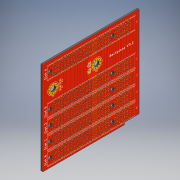
# Autodesk Inventor part: Backplane_PCB
Saved by Autodesk Inventor 2018 (Build 220112000, 112)
## iProperties
Created: 2018-10-18
Part Number: Backplane_PCB
Material: Epoxy Resin
Document SubType Name: Modeling
Designer: Bradley
Density: 1.14 g/cm^3
Appearance: Smooth - Dark Gray
Author: Bradley
Autodesk Inventor part; units mm, degrees
ref_plane "YZ Plane" through (0, 0, 0) normal (1, 0, 0) x (0, 1, 0)
ref_plane "XZ Plane" through (0, 0, 0) normal (0, 1, 0) x (-1, 0, 0)
ref_plane "XY Plane" through (0, 0, 0) normal (0, 0, 1) x (1, 0, 0)
sketch "Sketch11" plane through (0, 0, 0) normal (1, 0, 0) x (0, 1, 0)
  line L0 (-41.4, 41.6) -> (-32, 41.6)
  line L1 (-32, 41.6) -> (-32, 43)
  line L2 (-32, 43) -> (32, 43)
  line L3 (32, 43) -> (32, 41.6)
  line L4 (32, 41.6) -> (41.4, 41.6)
  line L5 (41.4, 41.6) -> (41.4, -41.6)
  line L6 (41.4, -41.6) -> (32, -41.6)
  line L7 (32, -41.6) -> (32, -43)
  line L8 (32, -43) -> (-32, -43)
  line L9 (-32, -43) -> (-32, -41.6)
  line L10 (-32, -41.6) -> (-41.4, -41.6)
  line L11 (-41.4, -41.6) -> (-41.4, 41.6)
  line L12 (41.4, 17) -> (-21, 17)
  line L13 (-21, 17) -> (-21, -43)
  point P0 (0, 0)
  point P1 (0, 43)
  point P2 (-41.4, 0)
  dimension "d86" = 83.2
  dimension "d87" = 9.4
  dimension "d88" = 82.8
  dimension "d89" = 86
  dimension "d149" = 21
  dimension "d150" = 17
  constraints: 28 end point, 9 perpendicular, 7 point on line, 3 collinear, 2 horizontal, 2 midpoint, 1 horizontal alignment, 1 vertical, 1 vertical alignment
  measures "d86" distance of L4.end L5.end
  measures "d87" distance of L3.end L4.end
  measures "d88" distance between parallel lines of L11 L5
  measures "d89" distance between parallel lines of L8 L2
  measures "d149" distance from line of point (0, 0) L13
  measures "d150" distance from line of point (0, 0) L12
extrude "Extrusion3" add sketch "Sketch11" along normal mid plane 1 contours L13 L12 L5 L6 L7 L8
fillet "Fillet2" radius 0.5 6 edges at (0, 32, -43) (0, 32, -41.6) (0, 41.4, -41.6) (0, -21, 17) (0, -21, -43) (0, 41.4, 17)
sketch "Sketch19" plane through (0.5, 0, 0) normal (1, 0, 0) x (0, 0, -1)
  line L0 (-17, -21.0036) -> (-17, 41.4036) construction
  line L1 (-17, 41.4036) -> (43, 41.4036) construction
  line L2 (43, 41.4036) -> (43, -21.0036) construction
  line L3 (43, -21.0036) -> (-17, -21.0036) construction
  line L4 (-17, 40.9) -> (-17, -20.5) projected
  line L5 (43, -20.5) -> (43, 31.5) projected
  point P0 (0, 0)
  point P1 (-17, 10.2)
  constraints: 2 collinear, 2 midpoint, 2 other
decal "Decal5"
sketch "Sketch20" plane through (-0.5, 0, 0) normal (-1, 0, 0) x (0, 0, 1)
  line L0 (17, 41.4036) -> (17, -21.0036) construction
  line L1 (17, -21.0036) -> (-43, -21.0036) construction
  line L2 (-43, -21.0036) -> (-43, 41.4036) construction
  line L3 (-43, 41.4036) -> (17, 41.4036) construction
  line L4 (17, -20.5) -> (17, 40.9) projected
  line L5 (-43, 31.5) -> (-43, -20.5) projected
  point P0 (0, 0)
  point P1 (17, 10.2)
  constraints: 2 collinear, 2 midpoint, 2 other
decal "Decal6"
sketch "Sketch14" plane through (0.5, 0, 0) normal (1, 0, 0) x (0, 0, -1)
  point P0 (0, 0)
  point P1 (0, -14)
  point P2 (0, 14)
  constraints: 2 other
hole "Hole7" at (0.5, -14, 0) at (0.5, 14, 0) direction (-1, 0, 0) diameter 3.3 end through all
sketch "Sketch15" plane through (0.5, 0, 0) normal (1, 0, 0) x (0, 0, -1)
  point P0 (0, 0)
  point P1 (37.5, 24)
  point P2 (37.5, -16.15)
  point P3 (28.5, 24)
  point P4 (28.5, -16.15)
  point P5 (19.5, 24)
  point P6 (19.5, -16.15)
  point P7 (10.5, 24)
  point P8 (10.5, -16.15)
  point P9 (-10.5, 24)
  point P10 (-10.5, -16.15)
  constraints: 10 other
hole "Hole8" at (0.5, 24, -37.5) at (0.5, -16.15, -37.5) at (0.5, 24, -28.5) at (0.5, -16.15, -28.5) at (0.5, 24, -19.5) at (0.5, -16.15, -19.5) at (0.5, 24, -10.5) at (0.5, -16.15, -10.5) at (0.5, 24, 10.5) at (0.5, -16.15, 10.5) direction (-1, 0, 0) diameter 2.35 end through all
sketch "Sketch16" plane through (0.5, 0, 0) normal (1, 0, 0) x (0, 0, -1)
  point P0 (0, 0)
  point P1 (40.75, 0.65)
  point P2 (36.25, 25.65)
  point P3 (34.25, 26.65)
  point P4 (40.75, 26.65)
  point P5 (38.75, 25.65)
  point P6 (36.25, 27.65)
  point P7 (34.25, 28.65)
  point P8 (40.75, 28.65)
  point P9 (38.75, 27.65)
  point P10 (36.25, 29.65)
  point P11 (34.25, 30.65)
  point P12 (40.75, 30.65)
  point P13 (38.75, 29.65)
  point P14 (36.25, 31.65)
  point P15 (34.25, 32.65)
  point P16 (40.75, 32.65)
  point P17 (38.75, 31.65)
  point P18 (36.25, 33.65)
  point P19 (34.25, 34.65)
  point P20 (40.75, 34.65)
  point P21 (38.75, 33.65)
  point P22 (36.25, 35.65)
  point P23 (38.75, 35.65)
  point P24 (34.25, 22.65)
  point P25 (40.75, 22.65)
  point P26 (38.75, 21.65)
  point P27 (36.25, 21.65)
  point P28 (34.25, 20.65)
  point P29 (40.75, 20.65)
  point P30 (38.75, 19.65)
  point P31 (36.25, 19.65)
  point P32 (34.25, 18.65)
  point P33 (40.75, 18.65)
  point P34 (38.75, 17.65)
  point P35 (36.25, 17.65)
  point P36 (34.25, 16.65)
  point P37 (40.75, 16.65)
  point P38 (38.75, 15.65)
  point P39 (36.25, 15.65)
  point P40 (34.25, 14.65)
  point P41 (40.75, 14.65)
  point P42 (38.75, 13.65)
  point P43 (36.25, 13.65)
  point P44 (34.25, 12.65)
  point P45 (40.75, 12.65)
  point P46 (38.75, 11.65)
  point P47 (36.25, 11.65)
  point P48 (34.25, 10.65)
  point P49 (40.75, 10.65)
  point P50 (38.75, 9.65)
  point P51 (36.25, 9.65)
  point P52 (34.25, 8.65)
  point P53 (40.75, 8.65)
  point P54 (38.75, 7.65)
  point P55 (36.25, 7.65)
  point P56 (34.25, 6.65)
  point P57 (40.75, 6.65)
  point P58 (38.75, 5.65)
  point P59 (36.25, 5.65)
  point P60 (34.25, 4.65)
  point P61 (40.75, 4.65)
  point P62 (38.75, 3.65)
  point P63 (36.25, 3.65)
  point P64 (34.25, 2.65)
  point P65 (40.75, 2.65)
  point P66 (38.75, 1.65)
  point P67 (36.25, 1.65)
  point P68 (34.25, 0.65)
  point P69 (38.75, -0.35)
  point P70 (36.25, -0.35)
  point P71 (34.25, -1.35)
  point P72 (40.75, -1.35)
  point P73 (38.75, -2.35)
  point P74 (36.25, -2.35)
  point P75 (34.25, -3.35)
  point P76 (40.75, -3.35)
  point P77 (38.75, -4.35)
  point P78 (36.25, -4.35)
  point P79 (34.25, -5.35)
  point P80 (40.75, -5.35)
  point P81 (38.75, -6.35)
  point P82 (36.25, -6.35)
  point P83 (34.25, -7.35)
  point P84 (40.75, -7.35)
  point P85 (38.75, -8.35)
  point P86 (36.25, -8.35)
  point P87 (34.25, -9.35)
  point P88 (40.75, -9.35)
  point P89 (38.75, -10.35)
  point P90 (36.25, -10.35)
  point P91 (34.25, -11.35)
  point P92 (40.75, -11.35)
  point P93 (38.75, -12.35)
  point P94 (36.25, -12.35)
  point P95 (34.25, -13.35)
  point P96 (40.75, -13.35)
  point P97 (38.75, -14.35)
  point P98 (36.25, -14.35)
  point P99 (27.25, 25.65)
  point P100 (25.25, 26.65)
  point P101 (31.75, 26.65)
  point P102 (29.75, 25.65)
  point P103 (27.25, 27.65)
  point P104 (25.25, 28.65)
  point P105 (31.75, 28.65)
  point P106 (29.75, 27.65)
  point P107 (27.25, 29.65)
  point P108 (25.25, 30.65)
  point P109 (31.75, 30.65)
  point P110 (29.75, 29.65)
  point P111 (27.25, 31.65)
  point P112 (25.25, 32.65)
  point P113 (31.75, 32.65)
  point P114 (29.75, 31.65)
  point P115 (27.25, 33.65)
  point P116 (25.25, 34.65)
  point P117 (31.75, 34.65)
  point P118 (29.75, 33.65)
  point P119 (27.25, 35.65)
  point P120 (29.75, 35.65)
  point P121 (25.25, 22.65)
  point P122 (31.75, 22.65)
  point P123 (29.75, 21.65)
  point P124 (27.25, 21.65)
  point P125 (25.25, 20.65)
  point P126 (31.75, 20.65)
  point P127 (29.75, 19.65)
  point P128 (27.25, 19.65)
  point P129 (25.25, 18.65)
  point P130 (31.75, 18.65)
  point P131 (29.75, 17.65)
  point P132 (27.25, 17.65)
  point P133 (25.25, 16.65)
  point P134 (31.75, 16.65)
  point P135 (29.75, 15.65)
  point P136 (27.25, 15.65)
  point P137 (25.25, 14.65)
  point P138 (31.75, 14.65)
  point P139 (29.75, 13.65)
  point P140 (27.25, 13.65)
  point P141 (25.25, 12.65)
  point P142 (31.75, 12.65)
  point P143 (29.75, 11.65)
  point P144 (27.25, 11.65)
  point P145 (25.25, 10.65)
  point P146 (31.75, 10.65)
  point P147 (29.75, 9.65)
  point P148 (27.25, 9.65)
  point P149 (25.25, 8.65)
  point P150 (31.75, 8.65)
  point P151 (29.75, 7.65)
  point P152 (27.25, 7.65)
  point P153 (25.25, 6.65)
  point P154 (31.75, 6.65)
  point P155 (29.75, 5.65)
  point P156 (27.25, 5.65)
  point P157 (25.25, 4.65)
  point P158 (31.75, 4.65)
  point P159 (29.75, 3.65)
  point P160 (27.25, 3.65)
  point P161 (25.25, 2.65)
  point P162 (31.75, 2.65)
  point P163 (29.75, 1.65)
  point P164 (27.25, 1.65)
  point P165 (25.25, 0.65)
  point P166 (31.75, 0.65)
  point P167 (29.75, -0.35)
  point P168 (27.25, -0.35)
  point P169 (25.25, -1.35)
  point P170 (31.75, -1.35)
  point P171 (29.75, -2.35)
  point P172 (27.25, -2.35)
  point P173 (25.25, -3.35)
  point P174 (31.75, -3.35)
  point P175 (29.75, -4.35)
  point P176 (27.25, -4.35)
  point P177 (25.25, -5.35)
  point P178 (31.75, -5.35)
  point P179 (29.75, -6.35)
  point P180 (27.25, -6.35)
  point P181 (25.25, -7.35)
  point P182 (31.75, -7.35)
  point P183 (29.75, -8.35)
  point P184 (27.25, -8.35)
  point P185 (25.25, -9.35)
  point P186 (31.75, -9.35)
  point P187 (29.75, -10.35)
  point P188 (27.25, -10.35)
  point P189 (25.25, -11.35)
  point P190 (31.75, -11.35)
  point P191 (29.75, -12.35)
  point P192 (27.25, -12.35)
  point P193 (25.25, -13.35)
  point P194 (31.75, -13.35)
  point P195 (29.75, -14.35)
  point P196 (27.25, -14.35)
  point P197 (18.25, 25.65)
  point P198 (16.25, 26.65)
  point P199 (22.75, 26.65)
  constraints: 490 other
hole "Hole9" at (0.5, 0.65, -40.75) at (0.5, 25.65, -36.25) at (0.5, 26.65, -34.25) at (0.5, 26.65, -40.75) at (0.5, 25.65, -38.75) at (0.5, 27.65, -36.25) at (0.5, 28.65, -34.25) at (0.5, 28.65, -40.75) at (0.5, 27.65, -38.75) at (0.5, 29.65, -36.25) at (0.5, 30.65, -34.25) at (0.5, 30.65, -40.75) at (0.5, 29.65, -38.75) at (0.5, 31.65, -36.25) at (0.5, 32.65, -34.25) at (0.5, 32.65, -40.75) at (0.5, 31.65, -38.75) at (0.5, 33.65, -36.25) at (0.5, 34.65, -34.25) at (0.5, 34.65, -40.75) at (0.5, 33.65, -38.75) at (0.5, 35.65, -36.25) at (0.5, 35.65, -38.75) at (0.5, 22.65, -34.25) at (0.5, 22.65, -40.75) at (0.5, 21.65, -38.75) at (0.5, 21.65, -36.25) at (0.5, 20.65, -34.25) at (0.5, 20.65, -40.75) at (0.5, 19.65, -38.75) at (0.5, 19.65, -36.25) at (0.5, 18.65, -34.25) at (0.5, 18.65, -40.75) at (0.5, 17.65, -38.75) at (0.5, 17.65, -36.25) at (0.5, 16.65, -34.25) at (0.5, 16.65, -40.75) at (0.5, 15.65, -38.75) at (0.5, 15.65, -36.25) at (0.5, 14.65, -34.25) at (0.5, 14.65, -40.75) at (0.5, 13.65, -38.75) at (0.5, 13.65, -36.25) at (0.5, 12.65, -34.25) at (0.5, 12.65, -40.75) at (0.5, 11.65, -38.75) at (0.5, 11.65, -36.25) at (0.5, 10.65, -34.25) at (0.5, 10.65, -40.75) at (0.5, 9.65, -38.75) direction (-1, 0, 0) diameter 0.7 end through all and at (0.5, 9.65, -36.25) (0.5, 8.65, -34.25) (0.5, 8.65, -40.75) (0.5, 7.65, -38.75) (0.5, 7.65, -36.25) (0.5, 6.65, -34.25) (0.5, 6.65, -40.75) (0.5, 5.65, -38.75) (0.5, 5.65, -36.25) (0.5, 4.65, -34.25) (0.5, 4.65, -40.75) (0.5, 3.65, -38.75) (0.5, 3.65, -36.25) (0.5, 2.65, -34.25) (0.5, 2.65, -40.75) (0.5, 1.65, -38.75) (0.5, 1.65, -36.25) (0.5, 0.65, -34.25) (0.5, -0.35, -38.75) (0.5, -0.35, -36.25) (0.5, -1.35, -34.25) (0.5, -1.35, -40.75) (0.5, -2.35, -38.75) (0.5, -2.35, -36.25) (0.5, -3.35, -34.25) (0.5, -3.35, -40.75) (0.5, -4.35, -38.75) (0.5, -4.35, -36.25) (0.5, -5.35, -34.25) (0.5, -5.35, -40.75) (0.5, -6.35, -38.75) (0.5, -6.35, -36.25) (0.5, -7.35, -34.25) (0.5, -7.35, -40.75) (0.5, -8.35, -38.75) (0.5, -8.35, -36.25) (0.5, -9.35, -34.25) (0.5, -9.35, -40.75) (0.5, -10.35, -38.75) (0.5, -10.35, -36.25) (0.5, -11.35, -34.25) (0.5, -11.35, -40.75) (0.5, -12.35, -38.75) (0.5, -12.35, -36.25) (0.5, -13.35, -34.25) (0.5, -13.35, -40.75) (0.5, -14.35, -38.75) (0.5, -14.35, -36.25) (0.5, 25.65, -27.25) (0.5, 26.65, -25.25) (0.5, 26.65, -31.75) (0.5, 25.65, -29.75) (0.5, 27.65, -27.25) (0.5, 28.65, -25.25) (0.5, 28.65, -31.75) (0.5, 27.65, -29.75) (0.5, 29.65, -27.25) (0.5, 30.65, -25.25) (0.5, 30.65, -31.75) (0.5, 29.65, -29.75) (0.5, 31.65, -27.25) (0.5, 32.65, -25.25) (0.5, 32.65, -31.75) (0.5, 31.65, -29.75) (0.5, 33.65, -27.25) (0.5, 34.65, -25.25) (0.5, 34.65, -31.75) (0.5, 33.65, -29.75) (0.5, 35.65, -27.25) (0.5, 35.65, -29.75) (0.5, 22.65, -25.25) (0.5, 22.65, -31.75) (0.5, 21.65, -29.75) (0.5, 21.65, -27.25) (0.5, 20.65, -25.25) (0.5, 20.65, -31.75) (0.5, 19.65, -29.75) (0.5, 19.65, -27.25) (0.5, 18.65, -25.25) (0.5, 18.65, -31.75) (0.5, 17.65, -29.75) (0.5, 17.65, -27.25) (0.5, 16.65, -25.25) (0.5, 16.65, -31.75) (0.5, 15.65, -29.75) (0.5, 15.65, -27.25) (0.5, 14.65, -25.25) (0.5, 14.65, -31.75) (0.5, 13.65, -29.75) (0.5, 13.65, -27.25) (0.5, 12.65, -25.25) (0.5, 12.65, -31.75) (0.5, 11.65, -29.75) (0.5, 11.65, -27.25) (0.5, 10.65, -25.25) (0.5, 10.65, -31.75) (0.5, 9.65, -29.75) (0.5, 9.65, -27.25) (0.5, 8.65, -25.25) (0.5, 8.65, -31.75) (0.5, 7.65, -29.75) (0.5, 7.65, -27.25) (0.5, 6.65, -25.25) (0.5, 6.65, -31.75) (0.5, 5.65, -29.75) (0.5, 5.65, -27.25) (0.5, 4.65, -25.25) (0.5, 4.65, -31.75) (0.5, 3.65, -29.75) (0.5, 3.65, -27.25) (0.5, 2.65, -25.25) (0.5, 2.65, -31.75) (0.5, 1.65, -29.75) (0.5, 1.65, -27.25) (0.5, 0.65, -25.25) (0.5, 0.65, -31.75) (0.5, -0.35, -29.75) (0.5, -0.35, -27.25) (0.5, -1.35, -25.25) (0.5, -1.35, -31.75) (0.5, -2.35, -29.75) (0.5, -2.35, -27.25) (0.5, -3.35, -25.25) (0.5, -3.35, -31.75) (0.5, -4.35, -29.75) (0.5, -4.35, -27.25) (0.5, -5.35, -25.25) (0.5, -5.35, -31.75) (0.5, -6.35, -29.75) (0.5, -6.35, -27.25) (0.5, -7.35, -25.25) (0.5, -7.35, -31.75) (0.5, -8.35, -29.75) (0.5, -8.35, -27.25) (0.5, -9.35, -25.25) (0.5, -9.35, -31.75) (0.5, -10.35, -29.75) (0.5, -10.35, -27.25) (0.5, -11.35, -25.25) (0.5, -11.35, -31.75) (0.5, -12.35, -29.75) (0.5, -12.35, -27.25) (0.5, -13.35, -25.25) (0.5, -13.35, -31.75) (0.5, -14.35, -29.75) (0.5, -14.35, -27.25) (0.5, 25.65, -18.25) (0.5, 26.65, -16.25) (0.5, 26.65, -22.75) (0.5, 25.65, -20.75) (0.5, 27.65, -18.25) (0.5, 28.65, -16.25) (0.5, 28.65, -22.75) (0.5, 27.65, -20.75) (0.5, 29.65, -18.25) (0.5, 30.65, -16.25) (0.5, 30.65, -22.75) (0.5, 29.65, -20.75) (0.5, 31.65, -18.25) (0.5, 32.65, -16.25) (0.5, 32.65, -22.75) (0.5, 31.65, -20.75) (0.5, 33.65, -18.25) (0.5, 34.65, -16.25) (0.5, 34.65, -22.75) (0.5, 33.65, -20.75) (0.5, 35.65, -18.25) (0.5, 35.65, -20.75) (0.5, 22.65, -16.25) (0.5, 22.65, -22.75) (0.5, 21.65, -20.75) (0.5, 21.65, -18.25) (0.5, 20.65, -16.25) (0.5, 20.65, -22.75) (0.5, 19.65, -20.75) (0.5, 19.65, -18.25) (0.5, 18.65, -16.25) (0.5, 18.65, -22.75) (0.5, 17.65, -20.75) (0.5, 17.65, -18.25) (0.5, 16.65, -16.25) (0.5, 16.65, -22.75) (0.5, 15.65, -20.75) (0.5, 15.65, -18.25) (0.5, 14.65, -16.25) (0.5, 14.65, -22.75) (0.5, 13.65, -20.75) (0.5, 13.65, -18.25) (0.5, 12.65, -16.25) (0.5, 12.65, -22.75) (0.5, 11.65, -20.75) (0.5, 11.65, -18.25) (0.5, 10.65, -16.25) (0.5, 10.65, -22.75) (0.5, 9.65, -20.75) (0.5, 9.65, -18.25) (0.5, 8.65, -16.25) (0.5, 8.65, -22.75) (0.5, 7.65, -20.75) (0.5, 7.65, -18.25) (0.5, 6.65, -16.25) (0.5, 6.65, -22.75) (0.5, 5.65, -20.75) (0.5, 5.65, -18.25) (0.5, 4.65, -16.25) (0.5, 4.65, -22.75) (0.5, 3.65, -20.75) (0.5, 3.65, -18.25) (0.5, 2.65, -16.25) (0.5, 2.65, -22.75) (0.5, 1.65, -20.75) (0.5, 1.65, -18.25) (0.5, 0.65, -16.25) (0.5, 0.65, -22.75) (0.5, -0.35, -20.75) (0.5, -0.35, -18.25) (0.5, -1.35, -16.25) (0.5, -1.35, -22.75) (0.5, -2.35, -20.75) (0.5, -2.35, -18.25) (0.5, -3.35, -16.25) (0.5, -3.35, -22.75) (0.5, -4.35, -20.75) (0.5, -4.35, -18.25) (0.5, -5.35, -16.25) (0.5, -5.35, -22.75) (0.5, -6.35, -20.75) (0.5, -6.35, -18.25) (0.5, -7.35, -16.25) (0.5, -7.35, -22.75) (0.5, -8.35, -20.75) (0.5, -8.35, -18.25) (0.5, -9.35, -16.25) (0.5, -9.35, -22.75) (0.5, -10.35, -20.75) (0.5, -10.35, -18.25) (0.5, -11.35, -16.25) (0.5, -11.35, -22.75) (0.5, -12.35, -20.75) (0.5, -12.35, -18.25) (0.5, -13.35, -16.25) (0.5, -13.35, -22.75) (0.5, -14.35, -20.75) (0.5, -14.35, -18.25) (0.5, 25.65, -9.25) (0.5, 26.65, -7.25) (0.5, 26.65, -13.75) (0.5, 25.65, -11.75) (0.5, 27.65, -9.25) (0.5, 28.65, -7.25) (0.5, 28.65, -13.75) (0.5, 27.65, -11.75) (0.5, 29.65, -9.25) (0.5, 30.65, -7.25) (0.5, 30.65, -13.75) (0.5, 29.65, -11.75) (0.5, 31.65, -9.25) (0.5, 32.65, -7.25) (0.5, 32.65, -13.75) (0.5, 31.65, -11.75) (0.5, 33.65, -9.25) (0.5, 34.65, -7.25) (0.5, 34.65, -13.75) (0.5, 33.65, -11.75) (0.5, 35.65, -9.25) (0.5, 35.65, -11.75) (0.5, 22.65, -7.25) (0.5, 22.65, -13.75) (0.5, 21.65, -11.75) (0.5, 21.65, -9.25) (0.5, 20.65, -7.25) (0.5, 20.65, -13.75) (0.5, 19.65, -11.75) (0.5, 19.65, -9.25) (0.5, 18.65, -7.25) (0.5, 18.65, -13.75) (0.5, 17.65, -11.75) (0.5, 17.65, -9.25) (0.5, 16.65, -7.25) (0.5, 16.65, -13.75) (0.5, 15.65, -11.75) (0.5, 15.65, -9.25) (0.5, 14.65, -7.25) (0.5, 14.65, -13.75) (0.5, 13.65, -11.75) (0.5, 13.65, -9.25) (0.5, 12.65, -7.25) (0.5, 12.65, -13.75) (0.5, 11.65, -11.75) (0.5, 11.65, -9.25) (0.5, 10.65, -7.25) (0.5, 10.65, -13.75) (0.5, 9.65, -11.75) (0.5, 9.65, -9.25) (0.5, 8.65, -7.25) (0.5, 8.65, -13.75) (0.5, 7.65, -11.75) (0.5, 7.65, -9.25) (0.5, 6.65, -7.25) (0.5, 6.65, -13.75) (0.5, 5.65, -11.75) (0.5, 5.65, -9.25) (0.5, 4.65, -7.25) (0.5, 4.65, -13.75) (0.5, 3.65, -11.75) (0.5, 3.65, -9.25) (0.5, 2.65, -7.25) (0.5, 2.65, -13.75) (0.5, 1.65, -11.75) (0.5, 1.65, -9.25) (0.5, 0.65, -7.25) (0.5, 0.65, -13.75) (0.5, -0.35, -11.75) (0.5, -0.35, -9.25) (0.5, -1.35, -7.25) (0.5, -1.35, -13.75) (0.5, -2.35, -11.75) (0.5, -2.35, -9.25) (0.5, -3.35, -7.25) (0.5, -3.35, -13.75) (0.5, -4.35, -11.75) (0.5, -4.35, -9.25) (0.5, -5.35, -7.25) (0.5, -5.35, -13.75) (0.5, -6.35, -11.75) (0.5, -6.35, -9.25) (0.5, -7.35, -7.25) (0.5, -7.35, -13.75) (0.5, -8.35, -11.75) (0.5, -8.35, -9.25) (0.5, -9.35, -7.25) (0.5, -9.35, -13.75) (0.5, -10.35, -11.75) (0.5, -10.35, -9.25) (0.5, -11.35, -7.25) (0.5, -11.35, -13.75) (0.5, -12.35, -11.75) (0.5, -12.35, -9.25) (0.5, -13.35, -7.25) (0.5, -13.35, -13.75) (0.5, -14.35, -11.75) (0.5, -14.35, -9.25) (0.5, 25.65, 11.75) (0.5, 26.65, 13.75) (0.5, 26.65, 7.25) (0.5, 25.65, 9.25) (0.5, 27.65, 11.75) (0.5, 28.65, 13.75) (0.5, 28.65, 7.25) (0.5, 27.65, 9.25) (0.5, 29.65, 11.75) (0.5, 30.65, 13.75) (0.5, 30.65, 7.25) (0.5, 29.65, 9.25) (0.5, 31.65, 11.75) (0.5, 32.65, 13.75) (0.5, 32.65, 7.25) (0.5, 31.65, 9.25) (0.5, 33.65, 11.75) (0.5, 34.65, 13.75) (0.5, 34.65, 7.25) (0.5, 33.65, 9.25) (0.5, 35.65, 11.75) (0.5, 35.65, 9.25) (0.5, 22.65, 13.75) (0.5, 22.65, 7.25) (0.5, 21.65, 9.25) (0.5, 21.65, 11.75) (0.5, 20.65, 13.75) (0.5, 20.65, 7.25) (0.5, 19.65, 9.25) (0.5, 19.65, 11.75) (0.5, 18.65, 13.75) (0.5, 18.65, 7.25) (0.5, 17.65, 9.25) (0.5, 17.65, 11.75) (0.5, 16.65, 13.75) (0.5, 16.65, 7.25) (0.5, 15.65, 9.25) (0.5, 15.65, 11.75) (0.5, 14.65, 13.75) (0.5, 14.65, 7.25) (0.5, 13.65, 9.25) (0.5, 13.65, 11.75) (0.5, 12.65, 13.75) (0.5, 12.65, 7.25) (0.5, 11.65, 9.25) (0.5, 11.65, 11.75) (0.5, 10.65, 13.75) (0.5, 10.65, 7.25) (0.5, 9.65, 9.25) (0.5, 9.65, 11.75) (0.5, 8.65, 13.75) (0.5, 8.65, 7.25) (0.5, 7.65, 9.25) (0.5, 7.65, 11.75) (0.5, 6.65, 13.75) (0.5, 6.65, 7.25) (0.5, 5.65, 9.25) (0.5, 5.65, 11.75) (0.5, 4.65, 13.75) (0.5, 4.65, 7.25) (0.5, 3.65, 9.25) (0.5, 3.65, 11.75) (0.5, 2.65, 13.75) (0.5, 2.65, 7.25) (0.5, 1.65, 9.25) (0.5, 1.65, 11.75) (0.5, 0.65, 13.75) (0.5, 0.65, 7.25) (0.5, -0.35, 9.25) (0.5, -0.35, 11.75) (0.5, -1.35, 13.75) (0.5, -1.35, 7.25) (0.5, -2.35, 9.25) (0.5, -2.35, 11.75) (0.5, -3.35, 13.75) (0.5, -3.35, 7.25) (0.5, -4.35, 9.25) (0.5, -4.35, 11.75) (0.5, -5.35, 13.75) (0.5, -5.35, 7.25) (0.5, -6.35, 9.25) (0.5, -6.35, 11.75) (0.5, -7.35, 13.75) (0.5, -7.35, 7.25) (0.5, -8.35, 9.25) (0.5, -8.35, 11.75) (0.5, -9.35, 13.75) (0.5, -9.35, 7.25) (0.5, -10.35, 9.25) (0.5, -10.35, 11.75) (0.5, -11.35, 13.75) (0.5, -11.35, 7.25) (0.5, -12.35, 9.25) (0.5, -12.35, 11.75) (0.5, -13.35, 13.75) (0.5, -13.35, 7.25) (0.5, -14.35, 9.25) (0.5, -14.35, 11.75)
sketch "Sketch21" plane through (0.5, 0, 0) normal (1, 0, 0) x (0, 0, -1)
  point P0 (0, 0)
  point P1 (0, 11.7)
  point P2 (-1.352, 12.139)
  point P3 (-2.187, 13.289)
  point P4 (-2.187, 14.711)
  point P5 (-1.352, 15.861)
  point P6 (0, 16.3)
  point P7 (1.352, 15.861)
  point P8 (2.187, 14.711)
  point P9 (2.187, 13.289)
  point P10 (1.352, 12.139)
  point P11 (0, -16.3)
  point P12 (-1.352, -15.861)
  point P13 (-2.187, -14.711)
  point P14 (-2.187, -13.289)
  point P15 (-1.352, -12.139)
  point P16 (0, -11.7)
  point P17 (1.352, -12.139)
  point P18 (2.187, -13.289)
  point P19 (2.187, -14.711)
  point P20 (1.352, -15.861)
  constraints: 21 other
hole "Hole12" at (0.5, 11.7, 0) at (0.5, 12.139, 1.352) at (0.5, 13.289, 2.187) at (0.5, 14.711, 2.187) at (0.5, 15.861, 1.352) at (0.5, 16.3, 0) at (0.5, 15.861, -1.352) at (0.5, 14.711, -2.187) at (0.5, 13.289, -2.187) at (0.5, 12.139, -1.352) at (0.5, -16.3, 0) at (0.5, -15.861, 1.352) at (0.5, -14.711, 2.187) at (0.5, -13.289, 2.187) at (0.5, -12.139, 1.352) at (0.5, -11.7, 0) at (0.5, -12.139, -1.352) at (0.5, -13.289, -2.187) at (0.5, -14.711, -2.187) at (0.5, -15.861, -1.352) direction (-1, 0, 0) diameter 0.45 end through all
sketch "Sketch22" plane through (0.5, 0, 0) normal (1, 0, 0) x (0, 0, -1)
  point P0 (0, 0)
  point P1 (0, -7.35)
  constraints: 1 other
hole "Hole13" at (0.5, -7.35, 0) direction (-1, 0, 0) diameter 0.3 end through all
body "Solid2"
